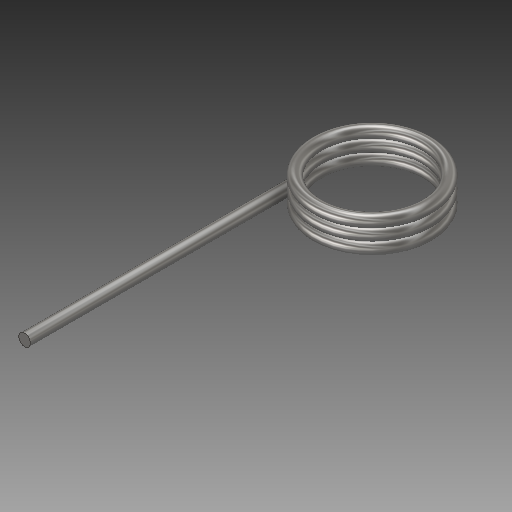
# Autodesk Inventor part: バネねじり270.z3
Saved by Autodesk Inventor 2020 (Build 240168000, 168)
## iProperties
Created: 2018-12-29
Part Number: バネねじり270.z3
Material: 鋼、炭素鋼
Document SubType Name: Modeling
Designer: 雪村
Density: 7.85 g/cm^3
Appearance: 半つや出し
Mass: 1.18313 g
Surface Area: 5.01353 cm^2
Volume: 0.150717 cm^3
Author: 雪村
Autodesk Inventor part; units mm, degrees
ref_plane "YZ Plane" through (0, 0, 0) normal (1, 0, 0) x (0, 1, 0)
ref_plane "XZ Plane" through (0, 0, 0) normal (0, 1, 0) x (-1, 0, 0)
ref_plane "XY Plane" through (0, 0, 0) normal (0, 0, 1) x (1, 0, 0)
sketch "スケッチ1" plane through (0, 0, 0) normal (0, 0, 1) x (1, 0, 0)
  circle A0 centre (-5.6, 0) radius 0.6
  line L0 (-5, 0) -> (-5, 0.9552) construction
  line L1 (0, 0) -> (0, 17.5733)
  circle A1 centre (-5.6, 1.2) radius 0.6
  circle A2 centre (-5.6, 2.4) radius 0.6
  dimension "d0" = 1.2
  dimension "d2" = 5
  dimension "d13" = 1.2
  dimension "d14" = 1.2
  constraints: 4 end point, 3 vertical, 2 centre point, 2 horizontal alignment, 2 vertical alignment, 1 equal radius, 3 other
  measures "d2" distance from line of L1.start L0
  measures "d13" diameter of A1
  measures "d14" diameter of A2
revolve "回転2" add sketch "スケッチ1" angle 360 about axis through (0, 0, 0) along (0, 1, 0)
sketch "スケッチ3" plane through (0, 0, 0) normal (0, 0, 1) x (1, 0, 0)
  arc A0 (-5.6, 0.6) -> (-5.6, -0.6) centre (-5.6, 0) ccw projected
  circle A1 centre (-5.6, 0) radius 0.6
  point P0 (0, 0)
  dimension "d16" = 1.2
  constraints: 1 centre point, 1 coincident
  measures "d16" diameter of A1
extrude "押し出し1" add sketch "スケッチ3" along normal blind 30
